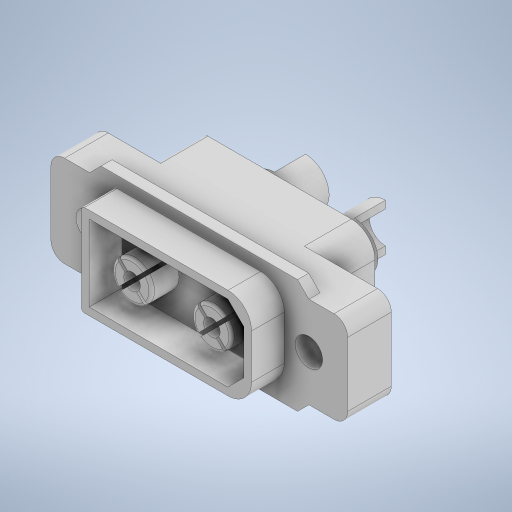
# Autodesk Inventor part: XT-60
Saved by Autodesk Inventor 2023 (Build 270158000, 158)
## iProperties
Created: 2023-11-22
Part Number: XT-60
Material: Generic
Document SubType Name: Modeling
Designer: LattePanda
Density: 1 g/cm^3
Appearance: Default
Author: LattePanda
Autodesk Inventor part; units mm, degrees
ref_plane "YZ Plane" through (0, 0, 0) normal (1, 0, 0) x (0, 1, 0)
ref_plane "XZ Plane" through (0, 0, 0) normal (0, 1, 0) x (-1, 0, 0)
ref_plane "XY Plane" through (0, 0, 0) normal (0, 0, 1) x (1, 0, 0)
sketch "Footprint" plane through (0, 0, 0) normal (0, 0, 1) x (1, 0, 0)
  circle A0 centre (-3.659, 0) radius 2.159
  circle A1 centre (3.659, 0) radius 2.159
  line L0 (-3.659, 0) -> (3.659, 0) construction
  line L1 (-1.5, 0) -> (1.5, 0) construction
  line L2 (-7.7851, 4.191) -> (7.7851, 4.191)
  line L3 (7.7851, 4.191) -> (7.7851, -4.191)
  line L4 (7.7851, -4.191) -> (-7.7851, -4.191)
  line L5 (-7.7851, -4.191) -> (-7.7851, 4.191)
  line L6 (-10.8991, 0) -> (10.8991, 0) construction
  line L7 (0, -5.8674) -> (0, 5.8674) construction
  point P0 (0, 0)
  point P1 (0, 0)
  point P2 (-7.7851, 0)
  point P3 (0, 4.191)
  dimension "d1" = 4.318
  dimension "d0" = 7.318
  dimension "d2" = 3
  dimension "d3" = 8.382
  dimension "d4" = 15.5702
  constraints: 12 end point, 4 point on line, 3 midpoint, 2 horizontal, 2 horizontal alignment, 2 parallel, 1 coincident, 1 perpendicular, 4 other
  measures "d0" distance of L0.start L0.end
  measures "d2" distance of L1.start L1.end
  measures "d3" distance of L2.end L3.end
  measures "d4" distance of L2.start L2.end
extrude "MountFeature" add sketch "Footprint" against normal blind 5.08 contours A0 | A1
extrude "Extrusion2" add sketch "Footprint" along normal blind 4.318 contours A0 | A1 | L2 L3 L4 L5
fillet "Fillet1" radius 2.159 2 edges at (7.7851, 4.191, 2.159) (7.7851, -4.191, 2.159)
fillet "Fillet2" radius 0.254 2 edges at (-7.7851, -4.191, 2.159) (-7.7851, 4.191, 2.159)
sketch "Sketch3" plane through (0, 0, 4.318) normal (0, 0, 1) x (1, 0, 0)
  line L0 (-13.6, 4.191) -> (13.6, 4.191)
  line L1 (13.6, 4.191) -> (13.6, -4.191)
  line L2 (13.6, -4.191) -> (-13.6, -4.191)
  line L3 (-13.6, -4.191) -> (-13.6, 4.191)
  line L4 (-25.1784, 0) -> (27.2051, 0) construction
  line L5 (0, -15.4188) -> (0, 16.666) construction
  line L6 (5.6261, 4.191) -> (-7.5311, 4.191) projected
  line L7 (-7.5311, -4.191) -> (5.6261, -4.191) projected
  circle A0 centre (10.05, 0) radius 1.25
  line L8 (13.6, 0) -> (11.3, 0) construction
  circle A1 centre (-10.05, 0) radius 1.25
  line L9 (-8.8, 0) -> (8.8, 0)
  point P0 (0, 0)
  point P1 (0, 4.191)
  point P2 (13.6, 0)
  dimension "d11" = 27.2
  dimension "d12" = 2.5
  dimension "d13" = 2.3
  dimension "d15" = 17.6
  constraints: 12 end point, 4 point on line, 3 collinear, 3 midpoint, 2 horizontal, 2 parallel, 2 point on circle, 1 centre point, 1 horizontal alignment, 1 perpendicular, 1 symmetric about line, 3 other
  measures "d11" distance of L0.start L0.end
  measures "d12" diameter of A0
  measures "d13" distance of point (13.6, 0) L8.end
  measures "d15" distance of L9.start L9.end
extrude "Extrusion3" add sketch "Sketch3" along normal blind 4
sketch "Sketch4" plane through (0, 0, 8.318) normal (0, 0, 1) x (1, 0, 0)
  circle A0 centre (3.659, 0) radius 2.159 projected
  circle A1 centre (-3.659, 0) radius 2.159 projected
  arc A2 (-7.5311, 4.191) -> (-7.7851, 3.937) centre (-7.5311, 3.937) ccw projected
  line L0 (5.6261, 4.191) -> (-7.5311, 4.191) projected
  arc A3 (7.7851, 2.032) -> (5.6261, 4.191) centre (5.6261, 2.032) ccw projected
  line L1 (7.7851, -2.032) -> (7.7851, 2.032) projected
  arc A4 (5.6261, -4.191) -> (7.7851, -2.032) centre (5.6261, -2.032) ccw projected
  line L2 (-7.5311, -4.191) -> (5.6261, -4.191) projected
  arc A5 (-7.7851, -3.937) -> (-7.5311, -4.191) centre (-7.5311, -3.937) ccw projected
  line L3 (-7.7851, 3.937) -> (-7.7851, -3.937) projected
  point P0 (0, 0)
extrude "Extrusion4" add sketch "Sketch4" along normal blind 3 contours A0 | A1 | L0 A3 L1 A4 L2 A5 L3 A2
sketch "Sketch5" plane through (0, 0, 11.318) normal (0, 0, 1) x (1, 0, 0)
  line L0 (-7.7851, 3.937) -> (-7.7851, -3.937) projected
  arc A0 (-7.7851, -3.937) -> (-7.5311, -4.191) centre (-7.5311, -3.937) ccw projected
  line L1 (-7.5311, -4.191) -> (5.6261, -4.191) projected
  arc A1 (5.6261, -4.191) -> (7.7851, -2.032) centre (5.6261, -2.032) ccw projected
  line L2 (7.7851, -2.032) -> (7.7851, 2.032) projected
  arc A2 (7.7851, 2.032) -> (5.6261, 4.191) centre (5.6261, 2.032) ccw projected
  line L3 (5.6261, 4.191) -> (-7.5311, 4.191) projected
  arc A3 (-7.5311, 4.191) -> (-7.7851, 3.937) centre (-7.5311, 3.937) ccw projected
  line L4 (-7.0851, 3.491) -> (5.6261, 3.491)
  arc A4 (7.0851, 2.032) -> (5.6261, 3.491) centre (5.6261, 2.032) ccw
  line L5 (7.0851, 2.032) -> (7.0851, -2.032)
  arc A5 (5.6261, -3.491) -> (7.0851, -2.032) centre (5.6261, -2.032) ccw
  line L6 (5.6261, -3.491) -> (-7.0851, -3.491)
  line L7 (-7.0851, -3.491) -> (-7.0851, 3.491)
  point P0 (0, 0)
  dimension "d20" = 0.7
  constraints: 8 end point, 4 point on circle, 2 centre point, 5 other
  measures "d20" distance between parallel lines of L3 L4
extrude "Extrusion5" cut sketch "Sketch5" against normal up to surface (3 mm away) contours L4 A4 L5 A5 L6 L7
sketch "Sketch6" plane through (-7.0851, 3.491, 8.318) normal (0, 0, 1) x (1, 0, 0)
  circle A0 centre (3.4261, -3.491) radius 2.159 construction
  circle A1 centre (10.7441, -3.491) radius 2.159 construction
  circle A2 centre (3.4261, -3.491) radius 1.8
  circle A3 centre (10.7441, -3.491) radius 1.8
  point P0 (7.0851, -3.491)
  dimension "d23" = 3.6
  constraints: 2 centre point, 2 coincident, 1 equal radius
  measures "d23" diameter of A2
extrude "Extrusion6" add sketch "Sketch6" along normal blind 2.5
sketch "Sketch7" plane through (-3.659, 0, 10.818) normal (0, 0, 1) x (1, 0, 0)
  circle A0 centre (0, 0) radius 1.8 construction
  circle A1 centre (7.318, 0) radius 1.8 construction
  circle A2 centre (0, 0) radius 0.75
  circle A3 centre (7.318, 0) radius 0.75
  point P0 (3.659, 0)
  dimension "d26" = 1.5
  dimension "d27" = 1.5
  constraints: 2 centre point, 2 coincident
  measures "d26" diameter of A2
  measures "d27" diameter of A3
extrude "Extrusion7" cut sketch "Sketch7" against normal up to surface (2.5 mm away)
fillet "Fillet3" radius 0.254 2 edges at (-5.459, 0, 10.818) (1.859, 0, 10.818)
sketch "Sketch8" plane through (3.659, 0, 10.818) normal (0, 0, 1) x (1, 0, 0)
  circle A0 centre (-7.318, 0) radius 1.8 construction
  circle A1 centre (-7.318, 0) radius 0.75 construction
  line L0 (-3.659, -5.8674) -> (-3.659, 5.8674) construction
  line L1 (-8.5908, -1.2728) -> (-6.0452, 1.2728) construction
  circle A2 centre (-7.318, 0) radius 1.8 projected
  line L2 (-8.4847, -1.3789) -> (-5.9391, 1.1667)
  line L3 (-6.1513, 1.3789) -> (-8.6969, -1.1667)
  arc A3 (-8.6969, -1.1667) -> (-8.4847, -1.3789) centre (-8.5908, -1.2728) ccw
  arc A4 (-5.9391, 1.1667) -> (-6.1513, 1.3789) centre (-6.0452, 1.2728) ccw
  line L4 (-7.318, 0) -> (-7.318, 1.8) construction
  line L5 (-6.1513, -1.3789) -> (-8.6969, 1.1667)
  line L6 (-8.4847, 1.3789) -> (-5.9391, -1.1667)
  arc A5 (-6.1513, -1.3789) -> (-5.9391, -1.1667) centre (-6.0452, -1.2728) ccw
  arc A6 (-8.4847, 1.3789) -> (-8.6969, 1.1667) centre (-8.5908, 1.2728) ccw
  line L7 (1.1667, -1.3789) -> (-1.3789, 1.1667)
  line L8 (-1.1667, 1.3789) -> (1.3789, -1.1667)
  arc A7 (1.1667, -1.3789) -> (1.3789, -1.1667) centre (1.2728, -1.2728) ccw
  arc A8 (-1.1667, 1.3789) -> (-1.3789, 1.1667) centre (-1.2728, 1.2728) ccw
  line L9 (1.1667, 1.3789) -> (-1.3789, -1.1667)
  arc A9 (1.3789, 1.1667) -> (1.1667, 1.3789) centre (1.2728, 1.2728) ccw
  line L10 (-1.1667, -1.3789) -> (1.3789, 1.1667)
  arc A10 (-1.3789, -1.1667) -> (-1.1667, -1.3789) centre (-1.2728, -1.2728) ccw
  point P0 (-3.659, 0)
  point P1 (0, -0.2121)
  point P2 (0.2121, 0)
  point P3 (0, 0.2121)
  point P4 (-0.2121, 0)
  point P5 (-7.1059, 0)
  point P6 (-7.318, 0.2121)
  point P7 (-7.5301, 0)
  point P8 (-7.318, -0.2121)
  dimension "d31" = 0.3
  dimension "d32" = 45
  constraints: 22 end point, 18 point on circle, 18 symmetric about line, 8 centre point, 4 tangent, 1 midpoint, 1 parallel, 1 vertical, 6 other
  measures "d31" diameter of A4
  measures "d32" angle of L4 L1
extrude "Extrusion8" cut sketch "Sketch8" against normal up to surface (2.5 mm away) contours L2 L6 L3 A2 | A2 L3 A4 L2 | L6 A5 L5 A2 | A2 L5 L2 L6 | L2 L5 L3 L6 | L6 L3 L5 A2 | A2 L5 A6 L6 | L2 A2 L3 L5 | L2 A3 L3 A2 | L7 L10 L8 A7 | L10 A10 L9 L7 | L7 L9 L8 L10 | L7 A8 L8 L9 | L8 L9 A9 L10
fillet "Fillet4" radius 1.25 4 edges at (13.6, -4.191, 6.318) (13.6, 4.191, 6.318) (-13.6, -4.191, 6.318) (-13.6, 4.191, 6.318)
sketch "Sketch9" plane through (0, 0, 11.318) normal (0, 0, 1) x (1, 0, 0)
  arc A0 (7.0851, 2.032) -> (5.6261, 3.491) centre (5.6261, 2.032) ccw projected
  arc A1 (5.6261, -3.491) -> (7.0851, -2.032) centre (5.6261, -2.032) ccw projected
  line L0 (-7.0851, 3.491) -> (5.6261, 3.491) projected
  line L1 (5.6261, 3.491) -> (7.0851, 2.032)
  line L2 (7.0851, 2.032) -> (7.0851, -2.032) projected
  arc A2 (5.6261, -3.491) -> (7.0851, -2.032) centre (5.6261, -2.032) ccw projected
  line L3 (7.0851, -2.032) -> (5.6261, -3.491)
  point P0 (0, 0)
  constraints: 4 end point, 1 perpendicular
extrude "Extrusion9" add sketch "Sketch9" against normal up to surface (3 mm away)
sketch "Sketch10" plane through (0, 0, 8.318) normal (0, 0, 1) x (1, 0, 0)
  circle A0 centre (-10.05, 0) radius 1.25 construction
  circle A1 centre (10.05, 0) radius 1.25 construction
  line L0 (-10.05, 0) -> (-10.05, 4.191) construction
  line L1 (-7.5311, 4.191) -> (-12.35, 4.191) construction
  line L2 (10.05, 0) -> (10.05, 4.191) construction
  line L3 (12.35, 4.191) -> (5.6261, 4.191) construction
  line L4 (10.05, 4.191) -> (0, 4.191)
  line L5 (5.6261, 4.191) -> (-7.5311, 4.191) projected
  line L6 (10.05, 4.191) -> (9.0113, 5.2297)
  line L7 (9.0113, 5.2297) -> (0, 5.2297)
  line L8 (0, 5.2297) -> (0, 4.191) construction
  line L9 (5.6261, 3.491) -> (7.0851, 2.032) projected
  line L10 (-10.05, 4.191) -> (0, 4.191)
  line L11 (-10.05, 4.191) -> (-9.0113, 5.2297)
  line L12 (-9.0113, 5.2297) -> (0, 5.2297)
  line L13 (-19.04, 0) -> (19.04, 0) construction
  line L14 (10.05, -4.191) -> (0, -4.191)
  line L15 (10.05, -4.191) -> (9.0113, -5.2297)
  line L16 (9.0113, -5.2297) -> (0, -5.2297)
  line L17 (-9.0113, -5.2297) -> (0, -5.2297)
  line L18 (-10.05, -4.191) -> (-9.0113, -5.2297)
  line L19 (-10.05, -4.191) -> (0, -4.191)
  point P0 (0, 0)
  constraints: 30 end point, 7 symmetric about line, 3 point on line, 2 vertical, 1 horizontal, 1 parallel, 1 perpendicular
extrude "Extrusion10" add sketch "Sketch10" against normal blind 1.02
sketch "Sketch11" plane through (3.659, 0, -5.08) normal (0, 0, -1) x (-1, 0, 0)
  circle A0 centre (0, 0) radius 2.159 projected
  circle A1 centre (0, 0) radius 1.459
  circle A2 centre (7.318, 0) radius 2.159 projected
  circle A3 centre (7.318, 0) radius 1.459
  point P0 (3.659, 0)
  dimension "d40" = 0.7
  dimension "d41" = 0.7
  constraints: 2 centre point
  measures "d40" radial gap between concentric circles of A0 A1
  measures "d41" radial gap between concentric circles of A2 A3
extrude "Extrusion11" cut sketch "Sketch11" against normal up to surface (5.08 mm away) contours A1 | A3
sketch "Sketch12" plane through (3.659, 0, -5.08) normal (0, 0, -1) x (-1, 0, 0)
  circle A0 centre (0, 0) radius 2.159 projected
  line L0 (0, -2.159) -> (0, 2.159)
  circle A1 centre (7.318, 0) radius 2.159 projected
  line L1 (7.318, -2.159) -> (7.318, 2.159)
  point P0 (3.659, 0)
  constraints: 4 end point, 4 point on circle, 2 coincident, 2 midpoint, 2 vertical
extrude "Extrusion12" cut sketch "Sketch12" against normal blind 2.85 contours L0 A0 | A1 L1 picked at (-0.5923, -0.4088) picked at (7.7667, 0.5627)
sketch "Sketch13" plane through (0, 0, 0) normal (0, 0, -1) x (-1, 0, 0)
  circle A0 centre (-3.659, 0) radius 2.159 projected
  circle A1 centre (3.659, 0) radius 2.159 projected
  arc A2 (7.7851, 3.937) -> (7.5311, 4.191) centre (7.5311, 3.937) ccw projected
  line L0 (-5.6261, 4.191) -> (7.5311, 4.191) projected
  arc A3 (-5.6261, 4.191) -> (-7.7851, 2.032) centre (-5.6261, 2.032) ccw projected
  line L1 (-7.7851, -2.032) -> (-7.7851, 2.032) projected
  arc A4 (-7.7851, -2.032) -> (-5.6261, -4.191) centre (-5.6261, -2.032) ccw projected
  line L2 (7.5311, -4.191) -> (-5.6261, -4.191) projected
  arc A5 (7.5311, -4.191) -> (7.7851, -3.937) centre (7.5311, -3.937) ccw projected
  line L3 (7.7851, 3.937) -> (7.7851, -3.937) projected
  arc A6 (-6.9851, -2.032) -> (-5.6261, -3.391) centre (-5.6261, -2.032) ccw
  line L4 (-6.9851, -2.032) -> (-6.9851, 2.032)
  arc A7 (-5.6261, 3.391) -> (-6.9851, 2.032) centre (-5.6261, 2.032) ccw
  line L5 (-5.6261, 3.391) -> (6.9851, 3.391)
  line L6 (6.9851, 3.391) -> (6.9851, -3.391)
  line L7 (6.9851, -3.391) -> (-5.6261, -3.391)
  point P0 (0, 0)
  dimension "d46" = 0.8
  constraints: 8 end point, 4 point on circle, 2 centre point, 5 other
  measures "d46" distance between parallel lines of L2 L7
extrude "Extrusion13" cut sketch "Sketch13" against normal blind 0.8 contours L4 A7 L5 L6 L7 A6
fillet "Fillet5" radius 0.254 2 edges at (-6.9851, -3.391, 0.4) (-6.9851, 3.391, 0.4)
equation "\"d41\" = d40"
body "Solid1"
